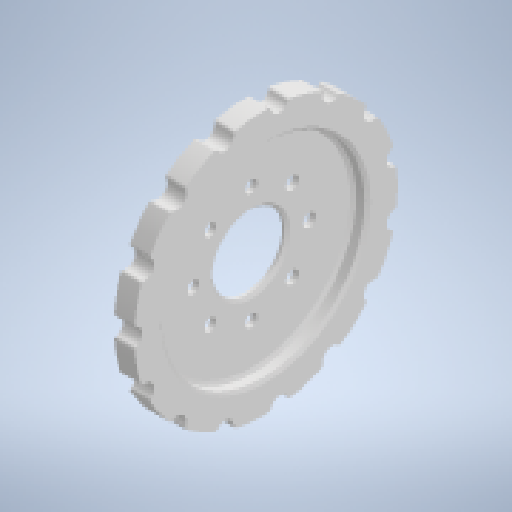
# Autodesk Inventor part: 主动外轮
Saved by Autodesk Inventor 2025.1 (Build 291241000, 241)
## iProperties
Created: 2025-08-27
Part Number: 主动外轮
Material: 常规
Document SubType Name: Modeling
Designer: Piw
Density: 1 g/cm^3
Appearance: 默认
Author: Piw
Autodesk Inventor part; units mm, degrees
ref_plane "YZ Plane" through (0, 0, 0) normal (1, 0, 0) x (0, 1, 0)
ref_plane "XZ Plane" through (0, 0, 0) normal (0, 1, 0) x (-1, 0, 0)
ref_plane "XY Plane" through (0, 0, 0) normal (0, 0, 1) x (1, 0, 0)
sketch "草图1" plane through (0, 0, 0) normal (1, 0, 0) x (0, 1, 0)
  circle A0 centre (0, 0) radius 46.5
  circle A1 centre (0, 0) radius 20 construction
  circle A2 centre (0, 0) radius 12.5
  circle A3 centre (20, 0) radius 2.1
  line L0 (20, 0) -> (0, 0) construction
  circle A4 centre (14.1421, 14.1421) radius 2.1
  circle A5 centre (0, 20) radius 2.1
  circle A6 centre (-14.1421, 14.1421) radius 2.1
  circle A7 centre (-20, 0) radius 2.1
  circle A8 centre (-14.1421, -14.1421) radius 2.1
  circle A9 centre (0, -20) radius 2.1
  circle A10 centre (14.1421, -14.1421) radius 2.1
  dimension "d1" = 40
  dimension "d0" = 93
  dimension "d2" = 25
  dimension "d3" = 4.2
  dimension "d6" = 360
  constraints: 10 centre point, 3 coincident, 2 end point, 1 horizontal, 1 horizontal alignment, 19 other
  measures "d0" diameter of A0
  measures "d2" diameter of A2
  measures "d3" diameter of A3
extrude "拉伸1" add sketch "草图1" along normal blind 7
sketch "草图2" plane through (7, 0, 0) normal (1, 0, 0) x (0, 0, -1)
  circle A0 centre (0, 0) radius 35
  dimension "d10" = 70
  constraints: 1 centre point, 1 coincident
  measures "d10" diameter of A0
extrude "拉伸2" cut sketch "草图2" against normal blind 5
chamfer "倒角1" distance 1 angle 45 2 edges at (7, 0, 35) (2, 0, 35)
sketch "草图3" plane through (7, 0, 0) normal (1, 0, 0) x (0, 0, -1)
  line L0 (0, 0) -> (43.1758, -9.1773) construction
  line L1 (0, 0) -> (45, 0) construction
  circle A0 centre (0, 0) radius 42.5 construction
  circle A1 centre (0, 0) radius 46.5 projected
  arc A2 (44.767, -12.5765) -> (46.012, -6.7192) centre (44.6035, -9.4808) ccw
  line L2 (47.7035, -9.4808) -> (47.7035, -3.4072)
  line L3 (42.5, 0) -> (42.5, -7.2037)
  circle A3 centre (44.6035, -9.4808) radius 1.55
  line L4 (44.6035, -9.4808) -> (43.959, -12.513) construction
  line L5 (43.959, -12.513) -> (44.7381, -12.6786)
  line L6 (45.2481, -6.4485) -> (46.0272, -6.6141)
  arc A4 (43.959, -12.513) -> (44.767, -12.5765) centre (44.6035, -9.4808) ccw construction
  arc A5 (45.2481, -6.4485) -> (43.959, -12.513) centre (44.6035, -9.4808) ccw
  arc A6 (46.012, -6.7192) -> (45.2481, -6.4485) centre (44.6035, -9.4808) ccw construction
  arc A7 (43.959, 12.513) -> (45.2481, 6.4485) centre (44.6035, 9.4808) ccw
  line L7 (45.2481, 6.4485) -> (46.0272, 6.6141)
  line L8 (43.959, 12.513) -> (44.7381, 12.6786)
  arc A8 (35.069, 29.311) -> (38.7133, 24.2951) centre (36.8912, 26.803) ccw
  line L9 (38.7133, 24.2951) -> (39.3577, 24.7633)
  line L10 (35.069, 29.311) -> (35.7135, 29.7792)
  arc A9 (20.1153, 41.0408) -> (25.4847, 37.9408) centre (22.8, 39.4908) ccw
  line L11 (25.4847, 37.9408) -> (25.883, 38.6306)
  line L12 (20.1153, 41.0408) -> (20.5136, 41.7306)
  arc A10 (1.6835, 45.6742) -> (7.8495, 45.0262) centre (4.7665, 45.3502) ccw
  line L13 (7.8495, 45.0262) -> (7.9328, 45.8183)
  line L14 (1.6835, 45.6742) -> (1.7667, 46.4664)
  arc A11 (-17.0395, 42.4102) -> (-11.1429, 44.3261) centre (-14.0912, 43.3682) ccw
  line L15 (-11.1429, 44.3261) -> (-11.389, 45.0837)
  line L16 (-17.0395, 42.4102) -> (-17.2856, 43.1678)
  arc A12 (-32.8161, 31.8131) -> (-28.2086, 35.9617) centre (-30.5124, 33.8874) ccw
  line L17 (-28.2086, 35.9617) -> (-28.7416, 36.5537)
  line L18 (-32.8161, 31.8131) -> (-33.3491, 32.4051)
  arc A13 (-42.9186, 15.7152) -> (-40.3968, 21.3792) centre (-41.6577, 18.5472) ccw
  line L19 (-40.3968, 21.3792) -> (-41.1245, 21.7032)
  line L20 (-42.9186, 15.7152) -> (-43.6462, 16.0392)
  arc A14 (-45.6, -3.1) -> (-45.6, 3.1) centre (-45.6, 0) ccw
  line L21 (-45.6, 3.1) -> (-46.3966, 3.1)
  line L22 (-45.6, -3.1) -> (-46.3966, -3.1)
  arc A15 (-40.3968, -21.3792) -> (-42.9186, -15.7152) centre (-41.6577, -18.5472) ccw
  line L23 (-42.9186, -15.7152) -> (-43.6462, -16.0392)
  line L24 (-40.3968, -21.3792) -> (-41.1245, -21.7032)
  arc A16 (-28.2086, -35.9617) -> (-32.8161, -31.8131) centre (-30.5124, -33.8874) ccw
  line L25 (-32.8161, -31.8131) -> (-33.3491, -32.4051)
  line L26 (-28.2086, -35.9617) -> (-28.7416, -36.5537)
  arc A17 (-11.1429, -44.3261) -> (-17.0395, -42.4102) centre (-14.0912, -43.3682) ccw
  line L27 (-17.0395, -42.4102) -> (-17.2856, -43.1678)
  line L28 (-11.1429, -44.3261) -> (-11.389, -45.0837)
  arc A18 (7.8495, -45.0262) -> (1.6835, -45.6742) centre (4.7665, -45.3502) ccw
  line L29 (1.6835, -45.6742) -> (1.7667, -46.4664)
  line L30 (7.8495, -45.0262) -> (7.9328, -45.8183)
  arc A19 (25.4847, -37.9408) -> (20.1153, -41.0408) centre (22.8, -39.4908) ccw
  line L31 (20.1153, -41.0408) -> (20.5136, -41.7306)
  line L32 (25.4847, -37.9408) -> (25.883, -38.6306)
  arc A20 (38.7133, -24.2951) -> (35.069, -29.311) centre (36.8912, -26.803) ccw
  line L33 (35.069, -29.311) -> (35.7135, -29.7792)
  line L34 (38.7133, -24.2951) -> (39.3577, -24.7633)
  point P0 (47.4355, 10.7417)
  point P1 (41.7557, 10.7054)
  point P2 (38.9655, 29.1068)
  point P3 (33.7914, 26.7635)
  point P4 (23.758, 42.439)
  point P5 (19.9843, 38.1938)
  point P6 (4.4425, 48.4332)
  point P7 (2.7218, 43.0202)
  point P8 (-15.6412, 46.0529)
  point P9 (-15.0114, 40.4079)
  point P10 (-33.0203, 35.7095)
  point P11 (-30.149, 30.8088)
  point P12 (-44.6899, 19.1917)
  point P13 (-40.0735, 15.8825)
  point P14 (-48.6323, -0.6445)
  point P15 (-43.069, -1.79)
  point P16 (-44.1656, -20.3693)
  point P17 (-38.6174, -19.153)
  point P18 (-32.0624, -36.5721)
  point P19 (-27.4886, -33.2042)
  point P20 (-14.4152, -46.4512)
  point P21 (-11.6067, -41.5142)
  point P22 (-43.6462, -16.0392)
  point P23 (-41.1245, -21.7032)
  point P24 (-17.2856, -43.1678)
  point P25 (-11.389, -45.0837)
  point P26 (-33.3491, -32.4051)
  point P27 (-28.7416, -36.5537)
  point P28 (-46.3966, 3.1)
  point P29 (-46.3966, -3.1)
  point P30 (-41.1245, 21.7032)
  point P31 (-43.6462, 16.0392)
  point P32 (-28.7416, 36.5537)
  point P33 (-33.3491, 32.4051)
  point P34 (-11.389, 45.0837)
  point P35 (-17.2856, 43.1678)
  point P36 (7.9328, 45.8183)
  point P37 (1.7667, 46.4664)
  point P38 (25.883, 38.6306)
  point P39 (20.5136, 41.7306)
  point P40 (39.3577, 24.7633)
  point P41 (35.7135, 29.7792)
  point P42 (46.0272, 6.6141)
  point P43 (44.7381, 12.6786)
  point P44 (5.7245, -48.2985)
  point P45 (6.2821, -42.646)
  point P46 (24.8743, -41.7945)
  point P47 (23.0847, -36.4039)
  point P48 (39.7232, -28.0639)
  point P49 (35.8957, -23.8672)
  point P50 (1.7667, -46.4664)
  point P51 (7.9328, -45.8183)
  point P52 (20.5136, -41.7306)
  point P53 (25.883, -38.6306)
  point P54 (35.7135, -29.7792)
  point P55 (39.3577, -24.7633)
  dimension "d17" = 85
  dimension "d16" = 12
  dimension "d27" = 3.1
  dimension "d28" = 3.1
  dimension "d31" = 360
  constraints: 70 end point, 69 point on circle, 19 centre point, 5 tangent, 3 perpendicular, 3 point on line, 2 coincident, 2 vertical, 1 horizontal, 1 horizontal alignment, 159 other
  measures "d16" angle of L1 L0
  measures "d27" diameter of A3
  measures "d28" radius of A5
extrude "拉伸3" cut sketch "草图3" against normal through all contours L7 A7 L8 A1 | A1 A3 L5 A5 L6 | A2 A1 A3 | L9 A8 L10 A1 | A3 A1 | A1 A3 | L11 A9 L12 A1 | A1 L33 A20 L34 | L13 A10 L14 A1 | A1 L31 A19 L32 | L15 A11 L16 A1 | A1 L29 A18 L30 | L17 A12 L18 A1 | A1 L27 A17 L28 | L19 A13 L20 A1 | A1 L25 A16 L26 | L21 A14 L22 A1 | A1 L23 A15 L24
chamfer "倒角2" distance 0.5 angle 45 30 edges at (3.5, -45.0837, 11.389) (3.5, -43.1678, 17.2856) (3.5, -36.5537, 28.7416) (3.5, -32.4051, 33.3491) (3.5, -21.7032, 41.1245) (3.5, -16.0392, 43.6462) (3.5, 3.1, 46.3966) (3.5, -3.1, 46.3966) (3.5, 16.0392, 43.6462) (3.5, 21.7032, 41.1245) (3.5, 32.4051, 33.3491) (3.5, 36.5537, 28.7416) (3.5, 43.1678, 17.2856) (3.5, 45.0837, 11.389) (3.5, 46.4664, -1.7667) (3.5, 45.8183, -7.9328) (3.5, 41.7306, -20.5136) (3.5, 38.6306, -25.883) (3.5, 29.7792, -35.7135) (3.5, 24.7633, -39.3577) (3.5, 12.6786, -44.7381) (3.5, 6.6141, -46.0272) (3.5, -6.6141, -46.0272) (3.5, -12.6786, -44.7381) (3.5, -29.7792, -35.7135) (3.5, -24.7633, -39.3577) (3.5, -38.6306, -25.883) (3.5, -41.7306, -20.5136) (3.5, -45.8183, -7.9328) (3.5, -46.4664, -1.7667)
chamfer "倒角3" distance 0.5 angle 45 82 edges at (0, 12.8668, -44.4242) (0, 6.3145, -45.8169) (0, -6.3145, -45.8169) (0, -12.8668, -44.4242) (0, -24.404, -39.2875) (0, -29.8234, -35.3501) (0, -38.2738, -25.9649) (0, -41.6232, -20.1636) (0, -45.5257, -8.1527) (0, -46.2259, -1.4907) (0, -44.9059, 11.0691) (0, -42.8358, 17.4399) (0, -36.5213, 28.377) (0, -32.039, 33.3551) (0, -21.822, 40.7782) (0, -15.7024, 43.5028) (0, -3.3494, 46.1285) (0, 3.3494, 46.1285) (0, 15.7024, 43.5028) (0, 21.822, 40.7782) (0, 32.039, 33.3551) (0, 36.5213, 28.377) (0, 42.8358, 17.4399) (0, 44.9059, 11.0691) (0, 45.5257, -8.1527) (0, 46.2259, -1.4907) (0, 38.2738, -25.9649) (0, 41.6232, -20.1636) (0, 29.8234, -35.3501) (0, 24.404, -39.2875) (0, 18.9133, -42.4799) (0, 34.5562, -31.1146) (0, 44.2241, -14.3693) (0, 46.2453, 4.8606) (0, 42.2672, -4.4425) (0, 45.1736, -7.865) (0, 45.8217, -1.699) (0, 40.4199, 13.1332) (0, 44.4671, 11.1887) (0, 42.5512, 17.0853) (0, 31.5837, 28.4381) (0, 36.0719, 28.3078) (0, 31.9233, 32.9153) (0, 17.2863, 38.8257) (0, 21.4395, 40.5322) (0, 15.7755, 43.054) (0, 0, 42.5) (0, 3.1, 45.7483) (0, -3.1, 45.7483) (0, -17.2863, 38.8257) (0, -15.7755, 43.054) (0, -21.4395, 40.5322) (0, -31.5837, 28.4381) (0, -31.9233, 32.9153) (0, -36.0719, 28.3078) (0, -40.4199, 13.1332) (0, -42.5512, 17.0853) (0, -44.4671, 11.1887) (0, -42.2672, -4.4425) (0, -45.8217, -1.699) (0, -45.1736, -7.865) (0, -36.8061, -21.25) (0, -41.1692, -20.1895) (0, -38.0692, -25.5588) (0, -18.9133, -42.4799) (0, -34.5562, -31.1146) (0, -24.9809, -34.3832) (0, -29.3981, -35.189) (0, -24.3822, -38.8333) (0, -8.8362, -41.5713) (0, -12.5439, -44.104) (0, -6.4793, -45.3931) (0, 0, -46.5) (0, 8.8362, -41.5713) (0, 6.4793, -45.3931) (0, 12.5439, -44.104) (0, 24.9809, -34.3832) (0, 24.3822, -38.8333) (0, 29.3981, -35.189) (0, 36.8061, -21.25) (0, 38.0692, -25.5588) (0, 41.1692, -20.1895)
sketch "草图4" plane through (7, 0, 0) normal (1, 0, 0) x (0, 0, -1)
  circle A0 centre (0, 0) radius 45.5
  circle A1 centre (0, 0) radius 50
  dimension "d41" = 100
  dimension "d42" = 91
  constraints: 2 centre point, 2 coincident
  measures "d41" diameter of A1
  measures "d42" diameter of A0
extrude "拉伸4" cut sketch "草图4" against normal blind 10
fillet "圆角1" radius 1 30 edges at (3.75, -35.8046, 28.0763) (3.75, -31.6651, 32.6737) (3.75, -21.2895, 40.212) (3.75, -15.6379, 42.7283) (3.75, -3.0932, 45.3947) (3.75, 3.0932, 45.3947) (3.75, 15.6379, 42.7283) (3.75, 21.2895, 40.212) (3.75, 35.8046, 28.0763) (3.75, 31.6651, 32.6737) (3.75, 42.2171, 16.9696) (3.75, 44.1288, 11.0859) (3.75, 45.4694, -1.6688) (3.75, 44.8227, -7.8213) (3.75, 40.8596, -20.0186) (3.75, 37.7664, -25.3762) (3.75, 29.1848, -34.907) (3.75, 24.1799, -38.5432) (3.75, 12.4637, -43.7596) (3.75, 6.4125, -45.0459) (3.75, -6.4125, -45.0459) (3.75, -12.4637, -43.7596) (3.75, -24.1799, -38.5432) (3.75, -29.1848, -34.907) (3.75, -37.7664, -25.3762) (3.75, -40.8596, -20.0186) (3.75, -44.8227, -7.8213) (3.75, -45.4694, -1.6688) (3.75, -44.1288, 11.0859) (3.75, -42.2171, 16.9696)
chamfer "倒角4" distance 1 angle 45 1 edges at (2, -12.5, 0)
